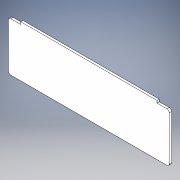
# Autodesk Inventor part: sides 3mm
Saved by Autodesk Inventor 2018.1 (Build 221171000, 171)
## iProperties
Created: 2018-11-28
Part Number: sides 3mm
Material: Aluminum 6061
Document SubType Name: Sheet Metal
Designer: RCCol
Density: 2.7 g/cm^3
Sheet Metal Rule: 3mm thick aluminum
Appearance: Aluminum - Flat
Author: RCCol
Autodesk Inventor part; units mm, degrees
ref_plane "YZ Plane" through (0, 0, 0) normal (1, 0, 0) x (0, 1, 0)
ref_plane "XZ Plane" through (0, 0, 0) normal (0, 1, 0) x (-1, 0, 0)
ref_plane "XY Plane" through (0, 0, 0) normal (0, 0, 1) x (1, 0, 0)
sketch "Sketch1" plane through (0, 0, 0) normal (0, 0, 1) x (1, 0, 0)
  line L0 (13.05, 69.85) -> (13.05, 66.85)
  line L1 (13.05, 66.85) -> (0, 66.85)
  arc A0 (0, 66.85) -> (-3, 63.85) centre (0, 63.85) ccw
  line L2 (-3, 63.85) -> (-3, 6)
  arc A1 (-3, 6) -> (0, 3) centre (0, 6) ccw
  line L3 (0, 3) -> (203.9, 3)
  arc A2 (203.9, 3) -> (206.9, 6) centre (203.9, 6) ccw
  line L4 (206.9, 6) -> (206.9, 63.85)
  arc A3 (206.9, 63.85) -> (203.9, 66.85) centre (203.9, 63.85) ccw
  line L5 (203.9, 66.85) -> (190.85, 66.85)
  line L6 (190.85, 66.85) -> (190.85, 69.85)
  line L7 (190.85, 69.85) -> (13.05, 69.85)
  line L8 (190.85, 66.85) -> (190.85, 69.85)
  line L9 (190.85, 66.85) -> (203.9, 66.85)
  line L10 (-3, 63.85) -> (-3, 6)
  line L11 (0, 3) -> (203.9, 3)
  line L12 (206.9, 6) -> (206.9, 63.85)
  arc A4 (203.9, 3) -> (206.9, 6) centre (203.9, 6) ccw
  line L13 (13.05, 66.85) -> (0, 66.85)
  line L14 (13.05, 66.85) -> (13.05, 69.85)
  point P0 (0, 0)
extrude "Plate1" add sketch "Sketch1" along normal blind 3
equation "\"d0\" = Thickness"
equation "\"BendRadius\" = Thickness"
equation "\"BendReliefWidth\" = Thickness"
equation "\"BendReliefDepth\" = 0.5 * Thickness"
equation "\"CornerReliefSize\" = 4 * Thickness"
equation "\"MinimumRemnant\" = 2 * Thickness"
equation "\"TransitionRadius\" = BendRadius"
equation "\"JacobiRadiusSize\" = BendRadius"
equation "\"GapSize\" = Thickness"
equation "\"Thickness\" = 3"
body "Solid1"
